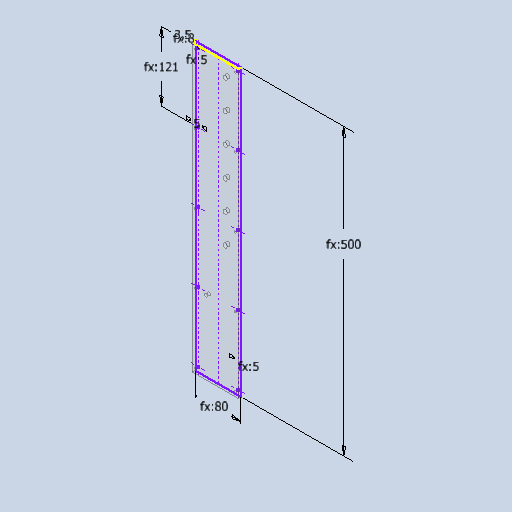
# Autodesk Inventor part: Back plate profile
Saved by Autodesk Inventor 2024 (Build 280153000, 153)
## iProperties
Created: 2021-11-04
Part Number: Back plate profile
Material: PMMA-Kunststoff
Document SubType Name: Modeling
Designer: espen
Density: 1.188 g/cm^3
Appearance: Polycarbonat - klar
Mass: 235.345 g
Surface Area: 863.681 cm^2
Volume: 198.102 cm^3
BackPlate_Width: 80,000 mm
Author: espen
Autodesk Inventor part; units mm, degrees
ref_plane "YZ Plane" through (0, 0, 0) normal (1, 0, 0) x (0, 1, 0)
ref_plane "XZ Plane" through (0, 0, 0) normal (0, 1, 0) x (-1, 0, 0)
sketch "Sketch1" plane through (0, 0, 0) normal (0, 0, 1) x (1, 0, 0)
  line L0 (0, 0) -> (80, 0)
  line L1 (80, 0) -> (80, 500)
  line L2 (80, 500) -> (0, 500)
  line L3 (0, 500) -> (0, 0)
  line L4 (40, 500) -> (40, 0) construction
  circle A0 centre (5, 492) radius 1.75 construction
  circle A1 centre (75, 492) radius 1.75 construction
  line L5 (5, 0) -> (5, 500) construction
  line L6 (75, 500) -> (75, 0) construction
  circle A2 centre (5, 371) radius 1.75 construction
  circle A3 centre (75, 371) radius 1.75 construction
  circle A4 centre (5, 250) radius 1.75 construction
  circle A5 centre (75, 250) radius 1.75 construction
  circle A6 centre (5, 129) radius 1.75 construction
  circle A7 centre (75, 129) radius 1.75 construction
  circle A8 centre (5, 8) radius 1.75 construction
  circle A9 centre (75, 8) radius 1.75 construction
  dimension "d0" = 500
  dimension "d2" = 3.5
  dimension "d5" = 5
  dimension "d6" = 8
  dimension "d13" = 5
  dimension "d14" = 5
  dimension "BackPlate_Width" = 80
  dimension "d20" = 121
  constraints: 14 end point, 10 centre point, 10 coincident, 4 point on line, 3 perpendicular, 2 midpoint, 2 parallel, 2 vertical, 1 horizontal, 1 symmetric about line, 17 other
  measures "d0" distance of L0.end L1.end
  measures "d2" diameter of A0
  measures "d5" distance from line of L3 A0.centre
  measures "d6" distance from line of L2 A0.centre
  measures "d13" distance between parallel lines of L3 L5
  measures "d14" distance between parallel lines of L1 L6
  measures "BackPlate_Width" distance between parallel lines of L1 L3
  measures "d20" distance of A0.centre A2.centre
extrude "Extrusion1" add sketch "Sketch1" along normal blind 5
hole "Bohrung1" at (5, 8, 0) at (75, 8, 0) at (75, 129, 0) at (5, 129, 0) at (5, 250, 0) at (75, 250, 0) at (5, 371, 0) at (75, 371, 0) at (5, 492, 0) at (75, 492, 0) direction (0, 0, 1) diameter 3.4 end through all clearance for "Inbusschraube DIN EN ISO 4762" size "M3" standard "DIN"
sketch "Skizze2" plane through (0, 0, 0) normal (0, 0, -1) x (-1, 0, 0)
  circle A0 centre (-23.75, 128.125) radius 2.75 projected
  circle A1 centre (-57.2, 220.3973) radius 3.75 projected
  circle A2 centre (-57.2, 271.2913) radius 3.75 projected
  circle A3 centre (-57.2, 322.1853) radius 3.75 projected
  circle A4 centre (-57.2, 373.0793) radius 3.75 projected
  circle A5 centre (-57.2, 423.9733) radius 3.75 projected
  circle A6 centre (-57.2, 474.8673) radius 3.75 projected
  point P0 (0, 0)
extrude "Extrusion2" cut sketch "Skizze2" against normal through all
sketch "Skizze3" plane through (0, 500, 0) normal (0, 1, 0) x (1, 0, 0)
  line L0 (80, 0) -> (0, 0) projected
  line L1 (0, 0) -> (0, -5) projected
  line L2 (80, -5) -> (0, -5) projected
  line L3 (80, 0) -> (80, -5) projected
  point P0 (0, 0)
ref_plane "Arbeitsebene1" through (71.8081, 420, 4.9726) normal (0, 1, 0) x (0, 0, 1)
equation "\"d0\" = GuidanceTrack_Length"
equation "\"d5\" = 0.5 * GuidanceTrac_OneSide_Thickness"
equation "\"d6\" = TopLit_Fixhole_Edge_Dist"
equation "\"d14\" = d13"
equation "\"BackPlate_Width\" = GuidanceTrac_Width"
equation "\"GuidanceTrack_Length\" = 500"
equation "\"GuidanceTrac_OneSide_Thickness\" = 10"
equation "\"TopLit_Fixhole_Edge_Dist\" = 8"
equation "\"GuidanceTrac_Width\" = 80"
body "Solid1"
